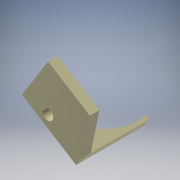
# Autodesk Inventor part: thumb_base_plate
Saved by Autodesk Inventor 2019 (Build 230136000, 136)
## iProperties
Created: 2024-08-27
Part Number: thumb_base_plate
Material: Nylon 6/6
Document SubType Name: Modeling
Designer: nic
Density: 1.13 g/cm^3
Appearance: Nylon 6
Author: nic
Autodesk Inventor part; units mm, degrees
ref_plane "YZ Plane" through (0, 0, 0) normal (1, 0, 0) x (0, 1, 0)
ref_plane "XZ Plane" through (0, 0, 0) normal (0, 1, 0) x (-1, 0, 0)
ref_plane "XY Plane" through (0, 0, 0) normal (0, 0, 1) x (1, 0, 0)
sketch "Skizze1" plane through (0, 0, 0) normal (0, 0, 1) x (1, 0, 0)
  circle A0 centre (0, 0) radius 0.5718 construction
  circle A1 centre (0, 0) radius 1.1
  line L0 (-3.4324, -5.4831) -> (-0.3524, -0.608) projected
  line L1 (12.1628, 19.8522) -> (1.5943, 2.5967) projected
  line L2 (0, 0) -> (-2.7013, -4.3259)
  line L3 (0, 0) -> (2.6665, 4.3474)
  line L4 (0, 0) -> (4.3474, -2.6665)
  line L5 (1.6594, -7.0489) -> (-6.9075, -1.6993)
  line L6 (-6.9075, -1.6993) -> (-1.5201, 6.9282)
  line L7 (-1.5201, 6.9282) -> (7.0468, 1.5787)
  line L8 (7.0468, 1.5787) -> (1.6594, -7.0489)
  dimension "d0" = 2.2
  dimension "d1" = 5.1
  dimension "d2" = 5.1
  dimension "d3" = 5.1
  dimension "d4" = 10.1
  constraints: 14 end point, 2 parallel, 2 point on line, 1 centre point, 1 coincident, 1 perpendicular
  measures "d0" diameter of A1
  measures "d1" distance of L2.start L2.end
  measures "d2" distance of L2.start L3.end
  measures "d3" distance of L2.start L4.end
  measures "d4" distance of L5.start L5.end
extrude "Extrusion1" add sketch "Skizze1" along normal blind 3 contours A1 L3 L1 L7 L8 L5 L0 | A1 L2 L5 L6 L7 L1 L3 | A1 L0 L2
sketch "Skizze2" plane through (0, 0, 0) normal (0, 0, -1) x (-1, 0, 0)
  circle A0 centre (0, 0) radius 1.1 projected
  line L0 (-1.6594, -7.0489) -> (6.9075, -1.6993) projected
  line L1 (6.9075, -1.6993) -> (1.5201, 6.9282) projected
  line L2 (1.5201, 6.9282) -> (-7.0468, 1.5787) projected
  line L3 (-7.0468, 1.5787) -> (-1.6594, -7.0489) projected
  circle A1 centre (0, 0) radius 1.1
  circle A2 centre (0.0269, 0) radius 2.5
  dimension "d7" = 5
  constraints: 2 centre point, 1 coincident, 1 concentric
  measures "d7" diameter of A2
extrude "Extrusion2" cut sketch "Skizze2" against normal blind 1 contours L3 L2 L1 L0
sketch "Skizze3" plane through (0, 0, 3) normal (0, 0, 1) x (1, 0, 0)
  circle A0 centre (0, 0) radius 1.1 projected
  line L0 (-6.9075, -1.6993) -> (1.6594, -7.0489) projected
  line L1 (1.6594, -7.0489) -> (7.0468, 1.5787) projected
  line L2 (7.0468, 1.5787) -> (-1.5201, 6.9282) projected
  line L3 (-1.5201, 6.9282) -> (-6.9075, -1.6993) projected
  line L4 (-2.6241, -4.3741) -> (-1.1, -1.79)
  line L5 (-6.9075, -1.6993) -> (1.6594, -7.0489)
  line L6 (1.6594, -7.0489) -> (3.2354, -4.5251)
  line L7 (3.2354, -4.5251) -> (-5.3316, 0.8245)
  line L8 (-5.3316, 0.8245) -> (-6.9075, -1.6993)
  dimension "d10" = 3
  constraints: 10 end point, 3 equal length, 1 midpoint, 1 perpendicular
  measures "d10" distance of L4.start L4.end
extrude "Extrusion3" cut sketch "Skizze3" against normal through all contours L3 L7 L4 L0 | L4 L7 L1 L0
sketch "Skizze4" plane through (0, 0, 3) normal (0, 0, 1) x (1, 0, 0)
  line L0 (-5.3316, 0.8245) -> (3.2354, -4.5251) projected
  line L1 (3.2354, -4.5251) -> (7.0468, 1.5787) projected
  line L2 (7.0468, 1.5787) -> (-1.5201, 6.9282) projected
  line L3 (-1.5201, 6.9282) -> (-5.3316, 0.8245) projected
  circle A0 centre (0, 0) radius 1.1 projected
  line L4 (-5.3316, 0.8245) -> (3.2354, -4.5251) projected
  line L5 (-5.3316, 0.8245) -> (3.2354, -4.5251)
  line L6 (3.2354, -4.5251) -> (8.5849, 4.0418)
  line L7 (8.5849, 4.0418) -> (0.018, 9.3914)
  line L8 (0.018, 9.3914) -> (-5.3316, 0.8245)
  dimension "d13" = 10.1
  constraints: 8 end point, 2 parallel, 2 point on line, 1 perpendicular
  measures "d13" distance of L6.end L5.end
extrude "Extrusion4" add sketch "Skizze4" against normal up to surface (2 mm away) contours L8 L7 L6 L2
sketch "Skizze5" plane through (0, 0, 3) normal (0, 0, 1) x (1, 0, 0)
  line L0 (4.2881, -6.9427) -> (6.1322, -4.0444) projected
  line L1 (5.7598, -3.8294) -> (4.7032, -3.2194) projected
  line L2 (-5.3316, 0.8245) -> (3.2354, -4.5251) projected
  line L3 (3.2354, -4.5251) -> (8.5849, 4.0418) projected
  line L4 (8.5849, 4.0418) -> (0.018, 9.3914) projected
  line L5 (0.018, 9.3914) -> (-5.3316, 0.8245) projected
  circle A0 centre (0, 0) radius 1.1 projected
  line L6 (3.2354, -4.5251) -> (8.5849, 4.0418) projected
  line L7 (3.2354, -4.5251) -> (4.2236, -2.9426)
  line L8 (4.2236, -2.9426) -> (7.6164, -5.0612)
  line L9 (7.6164, -5.0612) -> (6.6282, -6.6437)
  line L10 (6.6282, -6.6437) -> (3.2354, -4.5251)
  dimension "d16" = 4
  constraints: 8 end point, 2 parallel, 1 perpendicular, 1 point on line
  measures "d16" distance of L7.end L8.end
extrude "Extrusion5" add sketch "Skizze5" against normal blind 14 contours L10 L3 L8 L0 | L0 L8 L9 L10
sketch "Skizze6" plane through (7.6164, -5.0612, 3) normal (0.5296614, 0.8482092, 0) x (0.8482092, -0.5296614, 0)
  line L0 (-1.7975, 12.28) -> (-2.2192, 15.496) projected
  line L1 (-1.9046, 10.7265) -> (-1.9053, 12.2728) projected
  line L2 (-1.9046, 10.7265) -> (-2.6926, 7.736) projected
  line L3 (-2.2272, 9.066) -> (-3.4465, 6.126) projected
  line L4 (-4.252, 5.184) -> (-3.4465, 6.126) projected
  line L5 (-4, 2) -> (-4, 14) projected
  arc A0 (-4, 5.4787) -> (-2.0084, 13.888) centre (-13.8052, 12.2414) ccw construction
  arc A1 (-3.4465, 5.9662) -> (-1.8224, 14) centre (-13.8052, 12.2414) ccw
  line L6 (-4, 14) -> (0, 14) projected
  line L7 (-1.8224, 14) -> (-4, 14)
  line L8 (-4, 14) -> (-4, 5.1324)
  line L9 (-1.9018, 5.1324) -> (-1.8224, 5.1324)
  line L10 (-3.4465, 5.9662) -> (-4, 5.184)
  point P0 (-9.141, 3)
  constraints: 8 end point, 4 point on circle, 4 point on line, 2 centre point, 1 collinear, 1 midpoint, 1 parallel, 1 perpendicular, 1 tangent
extrude "Extrusion6" cut sketch "Skizze6" against normal through all
sketch "Skizze7" plane through (6.6282, -6.6437, 3) normal (0.8482092, -0.5296614, 0) x (0, 0, -1)
  line L0 (0, 0) -> (0, 1.8657) projected
  line L1 (0, 0) -> (14, 0) projected
  line L2 (14, 1.8657) -> (14, 0) projected
  line L3 (0, 1.8657) -> (14, 1.8657) projected
  point P0 (3, 2.1246)
extrude "Extrusion7" cut sketch "Skizze7" against normal blind 1
sketch "Skizze8" plane through (0, 0, 3) normal (0, 0, 1) x (1, 0, 0)
  circle A0 centre (0, 0) radius 1.1 projected
  line L0 (5.78, -6.1141) -> (6.7682, -4.5315) projected
  line L1 (6.7682, -4.5315) -> (4.2236, -2.9426) projected
  line L2 (4.2236, -2.9426) -> (8.5849, 4.0418) projected
  line L3 (8.5849, 4.0418) -> (0.018, 9.3914) projected
  line L4 (0.018, 9.3914) -> (-5.3316, 0.8245) projected
  line L5 (-5.3316, 0.8245) -> (5.78, -6.1141) projected
  line L6 (6.7682, -4.5315) -> (8.5849, 4.0418)
  constraints: 2 end point
extrude "Extrusion8" add sketch "Skizze8" against normal up to surface (2 mm away) contours L1 L2 L6
